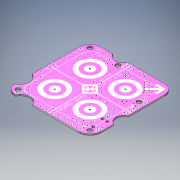
# Autodesk Inventor part: Eagle PCB rev 37
Saved by Autodesk Inventor 2016 (Build 200138000, 138)
## iProperties
Created: 2017-03-28
Part Number: Eagle PCB rev 37
Material: Generic
Document SubType Name: Modeling
Designer: Samuel Clay
Density: 1 g/cm^3
Appearance: Default
Author: Samuel Clay
Autodesk Inventor part; units mm, degrees
(part 1 of 2)
ref_plane "YZ Plane" through (0, 0, 0) normal (1, 0, 0) x (0, 1, 0)
ref_plane "XZ Plane" through (0, 0, 0) normal (0, 1, 0) x (-1, 0, 0)
ref_plane "XY Plane" through (0, 0, 0) normal (0, 0, 1) x (1, 0, 0)
sketch "PCB" plane through (0, 0, 0) normal (0, 0, 1) x (1, 0, 0)
  line L0 (-0.2705, -17.5177) -> (-0.2099, -17.5782)
  line L1 (0.0381, -17.435) -> (0.0159, -17.3523)
  line L2 (-0.2926, -17.435) -> (-0.2705, -17.5177)
  line L3 (-0.2099, -17.2918) -> (-0.2705, -17.3523)
  line L4 (-0.2705, -17.3523) -> (-0.2926, -17.435)
  line L5 (0.0159, -17.3523) -> (-0.0446, -17.2918)
  line L6 (-17.6003, -14.7625) -> (-17.5782, -14.8452)
  line L7 (-11.4091, 12.9967) -> (-11.4696, 12.9362)
  line L8 (-0.0446, -17.2918) -> (-0.1273, -17.2697)
  line L9 (-0.1273, -17.2697) -> (-0.2099, -17.2918)
  line L10 (-11.161, 12.8535) -> (-11.1832, 12.9362)
  line L11 (-0.2099, -17.5782) -> (-0.1273, -17.6003)
  line L12 (-11.2437, 12.9967) -> (-11.3264, 13.0189)
  line L13 (3.0162, 17.435) -> (3.0384, 17.3523)
  line L14 (-0.1273, -17.6003) -> (-0.0446, -17.5782)
  line L15 (-11.1832, 12.9362) -> (-11.2437, 12.9967)
  line L16 (-0.0446, -17.5782) -> (0.0159, -17.5177)
  line L17 (0.0159, -17.5177) -> (0.0381, -17.435)
  line L18 (-11.3264, 13.0189) -> (-11.4091, 12.9967)
  line L19 (-11.4696, 12.9362) -> (-11.4917, 12.8535)
  line L20 (-11.4917, 12.8535) -> (-11.4696, 12.7709)
  line L21 (-11.4696, 12.7709) -> (-11.4091, 12.7103)
  line L22 (-11.4091, 12.7103) -> (-11.3264, 12.6882)
  line L23 (-11.3264, 12.6882) -> (-11.2437, 12.7103)
  line L24 (-11.2437, 12.7103) -> (-11.1832, 12.7709)
  line L25 (-11.1832, 12.7709) -> (-11.161, 12.8535)
  line L26 (8.0176, -7.763) -> (7.9835, -7.6358)
  line L27 (7.9835, -7.6358) -> (7.8903, -7.5426)
  line L28 (7.8903, -7.5426) -> (7.763, -7.5085)
  line L29 (7.763, -7.5085) -> (7.6358, -7.5426)
  line L30 (7.6358, -7.5426) -> (7.5426, -7.6358)
  line L31 (7.5426, -7.6358) -> (7.5085, -7.763)
  line L32 (7.5085, -7.763) -> (7.5426, -7.8903)
  line L33 (7.5426, -7.8903) -> (7.6358, -7.9835)
  line L34 (7.6358, -7.9835) -> (7.763, -8.0176)
  line L35 (7.763, -8.0176) -> (7.8903, -7.9835)
  line L36 (7.8903, -7.9835) -> (7.9835, -7.8903)
  line L37 (7.9835, -7.8903) -> (8.0176, -7.763)
  line L38 (-18.2813, -15.6127) -> (-18.1967, -15.8611)
  line L39 (-13.3626, 15.4579) -> (-13.6171, 15.5261)
  line L40 (-6.9534, -18.4531) -> (13.3626, -18.4531)
  line L41 (-15.6051, -18.2836) -> (-15.3515, -18.3513)
  line L42 (14.9989, -18.1829) -> (15.3106, -18.0656)
  line L43 (-0.8082, 3.5474) -> (-0.7476, 3.6079)
  line L44 (-11.7528, 17.2918) -> (-11.6922, 17.3523)
  line L45 (-17.9797, -16.3387) -> (-17.8483, -16.5658)
  line L46 (16.719, -17.1898) -> (16.9621, -16.9621)
  line L47 (17.7711, -15.9078) -> (17.9281, -15.6141)
  line L48 (17.5782, -0.6809) -> (17.5177, -0.6204)
  line L49 (15.7965, -6.9168) -> (15.736, -6.8563)
  line L50 (17.5177, -0.6204) -> (17.435, -0.5982)
  line L51 (-14.2088, 17.2918) -> (-14.1262, 17.2697)
  line L52 (15.8187, -6.9995) -> (15.7965, -6.9168)
  line L53 (-13.983, 17.3523) -> (-13.9608, 17.435)
  line L54 (-14.2088, 17.5782) -> (-14.2694, 17.5177)
  line L55 (-14.2694, 17.5177) -> (-14.2915, 17.435)
  line L56 (-14.2915, 17.435) -> (-14.2694, 17.3523)
  line L57 (-14.2694, 17.3523) -> (-14.2088, 17.2918)
  line L58 (-0.7255, -15.3988) -> (-0.7476, -15.3161)
  line L59 (-13.983, 17.5177) -> (-14.0435, 17.5782)
  line L60 (-14.1262, 17.2697) -> (-14.0435, 17.2918)
  line L61 (-14.0435, 17.2918) -> (-13.983, 17.3523)
  line L62 (-14.1262, 17.6003) -> (-14.2088, 17.5782)
  line L63 (-13.9608, 17.435) -> (-13.983, 17.5177)
  line L64 (-14.0435, 17.5782) -> (-14.1262, 17.6003)
  line L65 (15.736, -6.8563) -> (15.6533, -6.8341)
  line L66 (-4.1997, -17.6003) -> (-4.117, -17.5782)
  line L67 (16.1624, -9.3283) -> (16.245, -9.3061)
  line L68 (17.435, -0.5982) -> (17.3523, -0.6204)
  line L69 (16.245, -9.3061) -> (16.3056, -9.2456)
  line L70 (-0.7476, -15.3161) -> (-0.8082, -15.2556)
  line L71 (-0.8082, -15.2556) -> (-0.8908, -15.2335)
  line L72 (-0.8908, -15.2335) -> (-0.9735, -15.2556)
  line L73 (-0.9735, -15.2556) -> (-1.034, -15.3161)
  line L74 (-1.034, -15.3161) -> (-1.0562, -15.3988)
  line L75 (-1.0562, -15.3988) -> (-1.034, -15.4815)
  line L76 (-1.034, -15.4815) -> (-0.9735, -15.542)
  line L77 (-0.9735, -15.542) -> (-0.8908, -15.5641)
  line L78 (-0.8908, -15.5641) -> (-0.8082, -15.542)
  line L79 (-0.8082, -15.542) -> (-0.7476, -15.4815)
  line L80 (-0.7476, -15.4815) -> (-0.7255, -15.3988)
  line L81 (8.1829, 15.1443) -> (8.1607, 15.2269)
  line L82 (-14.2375, 13.4453) -> (-14.298, 13.5058)
  line L83 (14.0435, -7.8744) -> (13.983, -7.9349)
  line L84 (13.983, -7.9349) -> (13.9608, -8.0176)
  line L85 (13.9608, -8.0176) -> (13.983, -8.1002)
  line L86 (13.983, -8.1002) -> (14.0435, -8.1607)
  line L87 (14.546, -10.8173) -> (14.5239, -10.7347)
  line L88 (14.5239, -10.7347) -> (14.4634, -10.6741)
  line L89 (14.2915, -8.0176) -> (14.2694, -7.9349)
  line L90 (14.4634, -10.6741) -> (14.3807, -10.652)
  line L91 (14.2694, -7.9349) -> (14.2088, -7.8744)
  line L92 (14.1262, -7.8522) -> (14.0435, -7.8744)
  line L93 (14.3807, -10.652) -> (14.298, -10.6741)
  line L94 (14.298, -10.6741) -> (14.2375, -10.7347)
  line L95 (14.2375, -10.7347) -> (14.2154, -10.8173)
  line L96 (14.2154, -10.8173) -> (14.2375, -10.9)
  line L97 (14.2375, -10.9) -> (14.298, -10.9605)
  line L98 (14.2088, -7.8744) -> (14.1262, -7.8522)
  line L99 (14.298, -10.9605) -> (14.3807, -10.9827)
  line L100 (14.0435, -8.1607) -> (14.1262, -8.1829)
  line L101 (14.3807, -10.9827) -> (14.4634, -10.9605)
  line L102 (14.4634, -10.9605) -> (14.5239, -10.9)
  line L103 (14.5239, -10.9) -> (14.546, -10.8173)
  line L104 (14.1262, -8.1829) -> (14.2088, -8.1607)
  line L105 (14.2088, -8.1607) -> (14.2694, -8.1002)
  line L106 (14.2694, -8.1002) -> (14.2915, -8.0176)
  line L107 (-14.298, 13.5058) -> (-14.3807, 13.5279)
  line L108 (-14.3807, 13.5279) -> (-14.4634, 13.5058)
  line L109 (13.5058, -15.0616) -> (13.4453, -15.0011)
  line L110 (16.3056, -0.5536) -> (16.245, -0.4931)
  line L111 (-18.4531, 13.3626) -> (-18.4531, -6.6988)
  line L112 (-17.7589, -7.0832) -> (-18.0967, -6.8742)
  line L113 (-16.8879, -7.8911) -> (-17.1517, -7.5941)
  line L114 (16.0192, -0.5536) -> (15.997, -0.6363)
  line L115 (-16.6541, -8.2122) -> (-16.8879, -7.8911)
  line L116 (-16.2848, -8.9145) -> (-16.4524, -8.5544)
  line L117 (-16.1527, -9.2892) -> (-16.2848, -8.9145)
  line L118 (16.245, -0.4931) -> (16.1624, -0.471)
  line L119 (-16.4524, -8.5544) -> (-16.6541, -8.2122)
  line L120 (2.5612, 11.9181) -> (2.5007, 11.9786)
  line L121 (-17.4429, -7.3239) -> (-17.7589, -7.0832)
  line L122 (-8.2721, 15.5943) -> (-8.0858, 15.7806)
  line L123 (-17.1517, -7.5941) -> (-17.4429, -7.3239)
  line L124 (-16.6541, -12.717) -> (-16.4524, -12.3748)
  line L125 (-8.0858, 15.7806) -> (-8.0176, 16.0351)
  line L126 (-18.0967, -6.8742) -> (-18.4531, -6.6988)
  line L127 (-16.0575, -9.6748) -> (-16.1527, -9.2892)
  line L128 (16.1624, -0.471) -> (16.0797, -0.4931)
  line L129 (-16, -10.0678) -> (-16.0575, -9.6748)
  line L130 (16.0797, -0.4931) -> (16.0192, -0.5536)
  line L131 (-15.9808, -10.4646) -> (-16, -10.0678)
  line L132 (-16, -10.8614) -> (-15.9808, -10.4646)
  line L133 (-8.0176, 13.9989) -> (-8.0858, 14.2534)
  line L134 (-16.0575, -11.2544) -> (-16, -10.8614)
  line L135 (-16.1527, -11.6401) -> (-16.0575, -11.2544)
  line L136 (15.997, -0.6363) -> (16.0192, -0.719)
  line L137 (-16.2848, -12.0147) -> (-16.1527, -11.6401)
  line L138 (-16.4524, -12.3748) -> (-16.2848, -12.0147)
  line L139 (16.0192, -0.719) -> (16.0797, -0.7795)
  line L140 (-8.9675, 14.2534) -> (-9.0357, 13.9989)
  line L141 (-16.8879, -13.0381) -> (-16.6541, -12.717)
  line L142 (16.0797, -0.7795) -> (16.1624, -0.8017)
  line L143 (-17.1517, -13.3351) -> (-16.8879, -13.0381)
  line L144 (-8.0858, 14.2534) -> (-8.2721, 14.4398)
  line L145 (-17.4429, -13.6053) -> (-17.1517, -13.3351)
  line L146 (16.3277, -0.6363) -> (16.3056, -0.5536)
  line L147 (16.1624, -0.8017) -> (16.245, -0.7795)
  line L148 (-17.7589, -13.846) -> (-17.4429, -13.6053)
  line L149 (-8.2721, 14.4398) -> (-8.5266, 14.508)
  line L150 (-18.0967, -14.055) -> (-17.7589, -13.846)
  line L151 (16.245, -0.7795) -> (16.3056, -0.719)
  line L152 (-18.4531, -14.2304) -> (-18.0967, -14.055)
  line L153 (15.6533, -6.8341) -> (15.5706, -6.8563)
  line L154 (16.3056, -0.719) -> (16.3277, -0.6363)
  line L155 (-18.4528, -14.5799) -> (-18.4354, -14.8417)
  line L156 (-8.5266, 14.508) -> (-8.7811, 14.4398)
  line L157 (-18.4354, -14.8417) -> (-18.4009, -15.1019)
  line L158 (-18.4009, -15.1019) -> (-18.3495, -15.3592)
  line L159 (-8.7811, 14.4398) -> (-8.9675, 14.2534)
  line L160 (-18.3495, -15.3592) -> (-18.2813, -15.6127)
  line L161 (-18.1967, -15.8611) -> (-18.096, -16.1034)
  line L162 (-18.096, -16.1034) -> (-17.9797, -16.3387)
  line L163 (-7.5426, 7.6358) -> (-7.5085, 7.763)
  line L164 (-9.1788, -14.8071) -> (-9.201, -14.8897)
  line L165 (-17.8483, -16.5658) -> (-17.7023, -16.7839)
  line L166 (-17.7023, -16.7839) -> (-17.5423, -16.9919)
  line L167 (-17.5423, -16.9919) -> (-17.3691, -17.1891)
  line L168 (-17.3691, -17.1891) -> (-17.1833, -17.3745)
  line L169 (-17.1833, -17.3745) -> (-16.9858, -17.5473)
  line L170 (-16.9858, -17.5473) -> (-16.7775, -17.7069)
  line L171 (-16.7775, -17.7069) -> (-16.5591, -17.8524)
  line L172 (-16.5591, -17.8524) -> (-16.3317, -17.9834)
  line L173 (-16.3317, -17.9834) -> (-16.0962, -18.0993)
  line L174 (-16.0962, -18.0993) -> (-15.8537, -18.1995)
  line L175 (-15.8537, -18.1995) -> (-15.6051, -18.2836)
  line L176 (-15.3515, -18.3513) -> (-15.0941, -18.4022)
  line L177 (-15.0941, -18.4022) -> (-14.8339, -18.4362)
  line L178 (-14.8339, -18.4362) -> (-14.572, -18.4531)
  line L179 (-14.572, -18.4531) -> (-14.4849, -18.4531)
  line L180 (-14.3095, -18.0967) -> (-14.4849, -18.4531)
  line L181 (-14.1005, -17.7589) -> (-14.3095, -18.0967)
  line L182 (-13.8598, -17.4429) -> (-14.1005, -17.7589)
  line L183 (-13.5897, -17.1517) -> (-13.8598, -17.4429)
  line L184 (-13.2927, -16.8879) -> (-13.5897, -17.1517)
  line L185 (-2.5898, 3.5474) -> (-2.5293, 3.6079)
  line L186 (-12.9715, -16.6541) -> (-13.2927, -16.8879)
  line L187 (-2.6725, 3.5253) -> (-2.5898, 3.5474)
  line L188 (-12.6293, -16.4524) -> (-12.9715, -16.6541)
  line L189 (-12.2692, -16.2848) -> (-12.6293, -16.4524)
  line L190 (-11.8946, -16.1527) -> (-12.2692, -16.2848)
  line L191 (-11.5089, -16.0575) -> (-11.8946, -16.1527)
  line L192 (-11.1159, -16) -> (-11.5089, -16.0575)
  line L193 (-10.7191, -15.9808) -> (-11.1159, -16)
  line L194 (-10.3224, -16) -> (-10.7191, -15.9808)
  line L195 (-9.9293, -16.0575) -> (-10.3224, -16)
  line L196 (-9.5437, -16.1527) -> (-9.9293, -16.0575)
  line L197 (-9.1691, -16.2848) -> (-9.5437, -16.1527)
  line L198 (-8.8089, -16.4524) -> (-9.1691, -16.2848)
  line L199 (-8.4667, -16.6541) -> (-8.8089, -16.4524)
  line L200 (-8.1456, -16.8879) -> (-8.4667, -16.6541)
  line L201 (-7.8486, -17.1517) -> (-8.1456, -16.8879)
  line L202 (-7.5785, -17.4429) -> (-7.8486, -17.1517)
  line L203 (-7.3378, -17.7589) -> (-7.5785, -17.4429)
  line L204 (-7.1287, -18.0967) -> (-7.3378, -17.7589)
  line L205 (-6.9534, -18.4531) -> (-7.1287, -18.0967)
  line L206 (13.3626, -18.4531) -> (13.6955, -18.4422)
  line L207 (13.6955, -18.4422) -> (14.027, -18.4095)
  line L208 (14.027, -18.4095) -> (14.3557, -18.3553)
  line L209 (14.3557, -18.3553) -> (14.6801, -18.2796)
  line L210 (14.6801, -18.2796) -> (14.9989, -18.1829)
  line L211 (15.3106, -18.0656) -> (15.6141, -17.9281)
  line L212 (15.6141, -17.9281) -> (15.9078, -17.7711)
  line L213 (15.9078, -17.7711) -> (16.1907, -17.5952)
  line L214 (16.1907, -17.5952) -> (16.4615, -17.4012)
  line L215 (16.4615, -17.4012) -> (16.719, -17.1898)
  line L216 (16.9621, -16.9621) -> (17.1898, -16.719)
  line L217 (17.1898, -16.719) -> (17.4012, -16.4615)
  line L218 (17.4012, -16.4615) -> (17.5952, -16.1907)
  line L219 (17.5952, -16.1907) -> (17.7711, -15.9078)
  line L220 (17.9281, -15.6141) -> (18.0656, -15.3106)
  line L221 (-2.5293, 3.6079) -> (-2.5072, 3.6906)
  line L222 (18.0656, -15.3106) -> (18.1829, -14.9989)
  line L223 (18.1829, -14.9989) -> (18.2796, -14.6801)
  line L224 (18.2796, -14.6801) -> (18.3553, -14.3557)
  line L225 (18.3553, -14.3557) -> (18.4095, -14.027)
  line L226 (18.4095, -14.027) -> (18.4422, -13.6955)
  line L227 (18.4422, -13.6955) -> (18.4531, -13.3626)
  line L228 (18.4531, -13.3626) -> (18.4531, -8.3763)
  line L229 (18.1449, -8.2246) -> (18.4531, -8.3763)
  line L230 (17.8528, -8.0438) -> (18.1449, -8.2246)
  line L231 (17.5795, -7.8357) -> (17.8528, -8.0438)
  line L232 (17.3276, -7.6021) -> (17.5795, -7.8357)
  line L233 (17.0995, -7.3452) -> (17.3276, -7.6021)
  line L234 (16.8973, -7.0675) -> (17.0995, -7.3452)
  line L235 (16.7229, -6.7715) -> (16.8973, -7.0675)
  line L236 (16.5779, -6.4601) -> (16.7229, -6.7715)
  line L237 (16.4637, -6.1361) -> (16.5779, -6.4601)
  line L238 (16.3813, -5.8026) -> (16.4637, -6.1361)
  line L239 (16.3316, -5.4627) -> (16.3813, -5.8026)
  line L240 (16.315, -5.1196) -> (16.3316, -5.4627)
  line L241 (16.3316, -4.7764) -> (16.315, -5.1196)
  line L242 (16.3813, -4.4365) -> (16.3316, -4.7764)
  line L243 (16.4637, -4.103) -> (16.3813, -4.4365)
  line L244 (16.5779, -3.779) -> (16.4637, -4.103)
  line L245 (16.7229, -3.4676) -> (16.5779, -3.779)
  line L246 (16.8973, -3.1716) -> (16.7229, -3.4676)
  line L247 (17.0995, -2.8939) -> (16.8973, -3.1716)
  line L248 (17.3276, -2.6371) -> (17.0995, -2.8939)
  line L249 (17.5795, -2.4035) -> (17.3276, -2.6371)
  line L250 (17.8528, -2.1953) -> (17.5795, -2.4035)
  line L251 (18.1449, -2.0145) -> (17.8528, -2.1953)
  line L252 (18.4531, -1.8628) -> (18.1449, -2.0145)
  line L253 (18.4531, -1.8628) -> (18.4531, 14.3807)
  line L254 (18.4531, 14.3807) -> (18.4444, 14.647)
  line L255 (18.4444, 14.647) -> (18.4183, 14.9122)
  line L256 (18.4183, 14.9122) -> (18.3748, 15.1752)
  line L257 (18.3748, 15.1752) -> (18.3143, 15.4347)
  line L258 (18.3143, 15.4347) -> (18.237, 15.6897)
  line L259 (18.237, 15.6897) -> (18.1431, 15.9391)
  line L260 (18.1431, 15.9391) -> (18.0331, 16.1819)
  line L261 (18.0331, 16.1819) -> (17.9075, 16.4169)
  line L262 (17.9075, 16.4169) -> (17.7668, 16.6432)
  line L263 (17.7668, 16.6432) -> (17.6116, 16.8598)
  line L264 (17.6116, 16.8598) -> (17.4425, 17.0658)
  line L265 (17.4425, 17.0658) -> (17.2603, 17.2603)
  line L266 (17.2603, 17.2603) -> (17.0658, 17.4425)
  line L267 (17.0658, 17.4425) -> (16.8598, 17.6116)
  line L268 (16.8598, 17.6116) -> (16.6432, 17.7668)
  line L269 (16.6432, 17.7668) -> (16.4169, 17.9075)
  line L270 (16.4169, 17.9075) -> (16.1819, 18.0331)
  line L271 (16.1819, 18.0331) -> (15.9391, 18.1431)
  line L272 (15.9391, 18.1431) -> (15.6897, 18.237)
  line L273 (15.6897, 18.237) -> (15.4347, 18.3143)
  line L274 (15.4347, 18.3143) -> (15.1752, 18.3749)
  line L275 (15.1752, 18.3749) -> (14.9122, 18.4183)
  line L276 (14.9122, 18.4183) -> (14.647, 18.4444)
  line L277 (14.647, 18.4444) -> (14.3807, 18.4531)
  line L278 (14.3807, 18.4531) -> (-1.6083, 18.4531)
  line L279 (-1.76, 18.1449) -> (-1.6083, 18.4531)
  line L280 (-1.9408, 17.8528) -> (-1.76, 18.1449)
  line L281 (-2.1489, 17.5795) -> (-1.9408, 17.8528)
  line L282 (-18.0656, 15.3106) -> (-18.1829, 14.9989)
  line L283 (-12.7103, 17.5177) -> (-12.7709, 17.5782)
  line L284 (-15.3988, -16.535) -> (-15.0261, -16.1624)
  line L285 (14.492, 2.3353) -> (14.5525, 2.2748)
  line L286 (16.026, -3.4361) -> (16.1624, -2.927)
  line L287 (-9.0357, 17.6003) -> (-9.1183, 17.5782)
  line L288 (1.8198, -17.435) -> (1.7976, -17.3523)
  line L289 (-17.5952, 16.1907) -> (-17.7711, 15.9078)
  line L290 (-14.6801, 18.2796) -> (-14.9989, 18.1829)
  line L291 (15.1443, -16.535) -> (15.6533, -16.6714)
  line L292 (-5.3291, 14.0816) -> (-5.3896, 14.1421)
  line L293 (15.6533, -16.6714) -> (16.1624, -16.535)
  line L294 (11.4696, 12.5163) -> (11.4917, 12.599)
  line L295 (16.1624, -16.535) -> (16.535, -16.1624)
  line L296 (-6.5731, 14.1102) -> (-6.4904, 14.0881)
  line L297 (16.535, -16.1624) -> (16.6714, -15.6533)
  line L298 (10.4196, 15.4815) -> (10.3975, 15.3988)
  line L299 (16.7828, 7.044) -> (16.8433, 6.9835)
  line L300 (-6.4904, 14.0881) -> (-6.4077, 14.1102)
  line L301 (10.7282, 15.3988) -> (10.706, 15.4815)
  line L302 (10.6455, 13.2513) -> (10.5628, 13.2734)
  line L303 (13.2194, 2.0808) -> (13.2799, 2.0203)
  line L304 (5.0996, 15.1443) -> (5.4723, 14.7716)
  line L305 (5.9813, 16.6714) -> (5.4723, 16.535)
  line L306 (5.4723, 16.535) -> (5.0996, 16.1624)
  line L307 (17.0691, 7.2094) -> (17.0086, 7.2699)
  line L308 (5.0996, 16.1624) -> (4.9632, 15.6533)
  line L309 (4.9632, 15.6533) -> (5.0996, 15.1443)
  line L310 (-6.6557, 14.2534) -> (-6.6336, 14.1708)
  line L311 (11.161, 12.599) -> (11.1832, 12.5163)
  line L312 (5.4723, 14.7716) -> (5.9813, 14.6352)
  line L313 (6.4904, 16.535) -> (5.9813, 16.6714)
  line L314 (5.9813, 14.6352) -> (6.4904, 14.7716)
  line L315 (-6.4904, 14.4188) -> (-6.5731, 14.3966)
  line L316 (6.4904, 14.7716) -> (6.8631, 15.1443)
  line L317 (10.4196, 13.0254) -> (10.4801, 12.9649)
  line L318 (6.9995, 15.6533) -> (6.8631, 16.1624)
  line L319 (6.8631, 15.1443) -> (6.9995, 15.6533)
  line L320 (10.706, 13.1907) -> (10.6455, 13.2513)
  line L321 (12.3286, 11.371) -> (12.3891, 11.3105)
  line L322 (12.4718, 11.619) -> (12.3891, 11.5968)
  line L323 (10.6455, 15.542) -> (10.5628, 15.5641)
  line L324 (10.4801, 12.9649) -> (10.5628, 12.9427)
  line L325 (11.2437, 12.7422) -> (11.1832, 12.6817)
  line L326 (11.4696, 12.6817) -> (11.4091, 12.7422)
  line L327 (13.2194, -17.3523) -> (13.1972, -17.435)
  line L328 (13.2799, -17.2918) -> (13.2194, -17.3523)
  line L329 (6.8631, 16.1624) -> (6.4904, 16.535)
  line L330 (11.4091, 12.4558) -> (11.4696, 12.5163)
  line L331 (4.117, 15.0011) -> (4.1997, 14.9789)
  line L332 (11.4917, 12.599) -> (11.4696, 12.6817)
  line L333 (11.3264, 12.4337) -> (11.4091, 12.4558)
  line L334 (-5.3896, 13.8557) -> (-5.3291, 13.9162)
  line L335 (11.2437, 12.4558) -> (11.3264, 12.4337)
  line L336 (-6.5731, 14.3966) -> (-6.6336, 14.3361)
  line L337 (4.3429, 15.2269) -> (4.2823, 15.2875)
  line L338 (13.3626, -17.2697) -> (13.2799, -17.2918)
  line L339 (-11.8354, 17.2697) -> (-11.7528, 17.2918)
  line L340 (-6.6336, 14.3361) -> (-6.6557, 14.2534)
  line L341 (4.3429, 15.0616) -> (4.365, 15.1443)
  line L342 (-5.3291, 13.9162) -> (-5.307, 13.9989)
  line L343 (-12.9362, 17.2918) -> (-12.8535, 17.2697)
  line L344 (-17.2697, -4.1997) -> (-17.2918, -4.117)
  line L345 (13.5279, -17.435) -> (13.5058, -17.3523)
  line L346 (13.5058, -17.3523) -> (13.4453, -17.2918)
  line L347 (-6.3472, 14.1708) -> (-6.3251, 14.2534)
  line L348 (17.0913, 7.1267) -> (17.0691, 7.2094)
  line L349 (-11.8354, 17.6003) -> (-11.9181, 17.5782)
  line L350 (-6.3472, 14.3361) -> (-6.4077, 14.3966)
  line L351 (10.7282, 13.1081) -> (10.706, 13.1907)
  line L352 (-5.555, 14.1421) -> (-5.6155, 14.0816)
  line L353 (16.8433, 7.2699) -> (16.7828, 7.2094)
  line L354 (17.0086, 7.2699) -> (16.9259, 7.2921)
  line L355 (-5.6155, 14.0816) -> (-5.6376, 13.9989)
  line L356 (11.4091, 12.7422) -> (11.3264, 12.7644)
  line L357 (-5.6155, 13.9162) -> (-5.555, 13.8557)
  line L358 (-6.4077, 14.3966) -> (-6.4904, 14.4188)
  line L359 (-5.3896, 14.1421) -> (-5.4723, 14.1642)
  line L360 (10.4196, 15.3161) -> (10.4801, 15.2556)
  line L361 (10.4801, 15.2556) -> (10.5628, 15.2335)
  line L362 (11.1832, 12.6817) -> (11.161, 12.599)
  line L363 (11.3264, 12.7644) -> (11.2437, 12.7422)
  line L364 (16.9259, 6.9614) -> (17.0086, 6.9835)
  line L365 (17.0691, 7.044) -> (17.0913, 7.1267)
  line L366 (10.4196, 13.1907) -> (10.3975, 13.1081)
  line L367 (12.6371, 11.4536) -> (12.6149, 11.5363)
  line L368 (10.3975, 13.1081) -> (10.4196, 13.0254)
  line L369 (13.2799, 2.0203) -> (13.3626, 1.9981)
  line L370 (16.8433, 6.9835) -> (16.9259, 6.9614)
  line L371 (17.0086, 6.9835) -> (17.0691, 7.044)
  line L372 (10.5628, 12.9427) -> (10.6455, 12.9649)
  line L373 (10.6455, 12.9649) -> (10.706, 13.0254)
  line L374 (10.706, 13.0254) -> (10.7282, 13.1081)
  line L375 (12.4718, 11.2883) -> (12.5544, 11.3105)
  line L376 (12.5544, 11.3105) -> (12.6149, 11.371)
  line L377 (12.6149, 11.371) -> (12.6371, 11.4536)
  line L378 (16.9259, 7.2921) -> (16.8433, 7.2699)
  line L379 (10.3975, 15.3988) -> (10.4196, 15.3161)
  line L380 (16.7606, 7.1267) -> (16.7828, 7.044)
  line L381 (10.5628, 15.2335) -> (10.6455, 15.2556)
  line L382 (10.6455, 15.2556) -> (10.706, 15.3161)
  line L383 (10.706, 15.3161) -> (10.7282, 15.3988)
  line L384 (10.706, 15.4815) -> (10.6455, 15.542)
  line L385 (4.0565, 15.2269) -> (4.0343, 15.1443)
  line L386 (10.5628, 15.5641) -> (10.4801, 15.542)
  line L387 (10.4801, 15.542) -> (10.4196, 15.4815)
  line L388 (4.0343, 15.1443) -> (4.0565, 15.0616)
  line L389 (4.0565, 15.0616) -> (4.117, 15.0011)
  line L390 (12.3286, 11.5363) -> (12.3064, 11.4536)
  line L391 (12.3064, 11.4536) -> (12.3286, 11.371)
  line L392 (12.3891, 11.3105) -> (12.4718, 11.2883)
  line L393 (11.7241, 14.4634) -> (11.6636, 14.5239)
  line L394 (11.6636, 14.5239) -> (11.5809, 14.546)
  line L395 (11.4377, 14.298) -> (11.4982, 14.2375)
  line L396 (11.5809, 14.546) -> (11.4982, 14.5239)
  line L397 (11.4982, 14.5239) -> (11.4377, 14.4634)
  line L398 (3.0384, 1.699) -> (3.0989, 1.6385)
  line L399 (-6.3251, 14.2534) -> (-6.3472, 14.3361)
  line L400 (11.4377, 14.4634) -> (11.4156, 14.3807)
  line L401 (11.4156, 14.3807) -> (11.4377, 14.298)
  line L402 (11.7463, 14.3807) -> (11.7241, 14.4634)
  line L403 (11.4982, 14.2375) -> (11.5809, 14.2154)
  line L404 (11.5809, 14.2154) -> (11.6636, 14.2375)
  line L405 (11.6636, 14.2375) -> (11.7241, 14.298)
  line L406 (11.7241, 14.298) -> (11.7463, 14.3807)
  line L407 (12.6371, 13.4899) -> (12.6149, 13.5725)
  line L408 (16.7828, 7.2094) -> (16.7606, 7.1267)
  line L409 (-2.5007, 14.9057) -> (-2.5612, 14.8452)
  line L410 (4.1997, 14.9789) -> (4.2823, 15.0011)
  line L411 (12.6149, 13.5725) -> (12.5544, 13.633)
  line L412 (12.5544, 13.633) -> (12.4718, 13.6552)
  line L413 (4.117, 15.2875) -> (4.0565, 15.2269)
  line L414 (12.4718, 13.6552) -> (12.3891, 13.633)
  line L415 (12.3891, 13.633) -> (12.3286, 13.5725)
  line L416 (12.3286, 13.5725) -> (12.3064, 13.4899)
  line L417 (4.1997, 15.3096) -> (4.117, 15.2875)
  line L418 (3.1816, 1.947) -> (3.0989, 1.9249)
  line L419 (12.3064, 13.4899) -> (12.3286, 13.4072)
  line L420 (4.2823, 15.2875) -> (4.1997, 15.3096)
  line L421 (12.3286, 13.4072) -> (12.3891, 13.3467)
  line L422 (12.3891, 13.3467) -> (12.4718, 13.3245)
  line L423 (12.4718, 13.3245) -> (12.5544, 13.3467)
  line L424 (12.5544, 13.3467) -> (12.6149, 13.4072)
  line L425 (12.6149, 13.4072) -> (12.6371, 13.4899)
  line L426 (12.3891, 11.5968) -> (12.3286, 11.5363)
  line L427 (13.1972, -17.435) -> (13.2194, -17.5177)
  line L428 (4.365, 15.1443) -> (4.3429, 15.2269)
  line L429 (3.0989, 1.6385) -> (3.1816, 1.6163)
  line L430 (3.1816, 1.6163) -> (3.2642, 1.6385)
  line L431 (13.2194, -17.5177) -> (13.2799, -17.5782)
  line L432 (8.5712, -14.0148) -> (8.6539, -14.037)
  line L433 (13.2799, -17.5782) -> (13.3626, -17.6003)
  line L434 (13.3626, -17.6003) -> (13.4453, -17.5782)
  line L435 (13.4453, -17.5782) -> (13.5058, -17.5177)
  line L436 (13.5058, -17.5177) -> (13.5279, -17.435)
  line L437 (8.5107, -13.9543) -> (8.5712, -14.0148)
  line L438 (-2.3353, 14.9057) -> (-2.418, 14.9278)
  line L439 (13.4453, -17.2918) -> (13.3626, -17.2697)
  line L440 (-2.3353, 14.6193) -> (-2.2748, 14.6798)
  line L441 (-2.418, 14.9278) -> (-2.5007, 14.9057)
  line L442 (-2.2527, 14.7625) -> (-2.2748, 14.8452)
  line L443 (8.7971, -13.9543) -> (8.8192, -13.8716)
  line L444 (8.7365, -14.0148) -> (8.7971, -13.9543)
  line L445 (11.2372, -17.435) -> (11.215, -17.3523)
  line L446 (11.215, -17.3523) -> (11.1545, -17.2918)
  line L447 (11.1545, -17.2918) -> (11.0719, -17.2697)
  line L448 (8.5107, -13.789) -> (8.4885, -13.8716)
  line L449 (10.9287, -17.5177) -> (10.9892, -17.5782)
  line L450 (11.0719, -17.2697) -> (10.9892, -17.2918)
  line L451 (8.8192, -13.8716) -> (8.7971, -13.789)
  line L452 (10.9892, -17.2918) -> (10.9287, -17.3523)
  line L453 (10.9287, -17.3523) -> (10.9065, -17.435)
  line L454 (10.9065, -17.435) -> (10.9287, -17.5177)
  line L455 (10.9892, -17.5782) -> (11.0719, -17.6003)
  line L456 (-2.2748, 14.8452) -> (-2.3353, 14.9057)
  line L457 (11.0719, -17.6003) -> (11.1545, -17.5782)
  line L458 (8.4885, -13.8716) -> (8.5107, -13.9543)
  line L459 (11.1545, -17.5782) -> (11.215, -17.5177)
  line L460 (8.7365, -13.7285) -> (8.6539, -13.7063)
  line L461 (11.215, -17.5177) -> (11.2372, -17.435)
  line L462 (8.9243, -17.5177) -> (8.9465, -17.435)
  line L463 (-2.418, 14.5971) -> (-2.3353, 14.6193)
  line L464 (-2.2748, 14.6798) -> (-2.2527, 14.7625)
  line L465 (8.5712, -13.7285) -> (8.5107, -13.789)
  line L466 (-2.5612, 14.6798) -> (-2.5007, 14.6193)
  line L467 (-2.5007, 14.6193) -> (-2.418, 14.5971)
  line L468 (8.9465, -17.435) -> (8.9243, -17.3523)
  line L469 (8.9243, -17.3523) -> (8.8638, -17.2918)
  line L470 (8.6539, -14.037) -> (8.7365, -14.0148)
  line L471 (8.8638, -17.2918) -> (8.7811, -17.2697)
  line L472 (8.7811, -17.2697) -> (8.6985, -17.2918)
  line L473 (8.6985, -17.2918) -> (8.6379, -17.3523)
  line L474 (-7.6358, 7.5426) -> (-7.5426, 7.6358)
  line L475 (8.6379, -17.3523) -> (8.6158, -17.435)
  line L476 (8.6539, -13.7063) -> (8.5712, -13.7285)
  line L477 (8.6158, -17.435) -> (8.6379, -17.5177)
  line L478 (8.6379, -17.5177) -> (8.6985, -17.5782)
  line L479 (8.6985, -17.5782) -> (8.7811, -17.6003)
  line L480 (8.7811, -17.6003) -> (8.8638, -17.5782)
  line L481 (8.8638, -17.5782) -> (8.9243, -17.5177)
  line L482 (8.7971, -13.789) -> (8.7365, -13.7285)
  line L483 (-2.5833, 14.7625) -> (-2.5612, 14.6798)
  line L484 (-2.5612, 14.8452) -> (-2.5833, 14.7625)
  line L485 (-4.0343, -17.435) -> (-4.0565, -17.3523)
  line L486 (-4.0565, -17.3523) -> (-4.117, -17.2918)
  line L487 (-4.117, -17.2918) -> (-4.1997, -17.2697)
  line L488 (-4.1997, -17.2697) -> (-4.2823, -17.2918)
  line L489 (-4.3429, -17.5177) -> (-4.2823, -17.5782)
  line L490 (-4.2823, -17.2918) -> (-4.3429, -17.3523)
  line L491 (-4.3429, -17.3523) -> (-4.365, -17.435)
  line L492 (-4.365, -17.435) -> (-4.3429, -17.5177)
  line L493 (-4.2823, -17.5782) -> (-4.1997, -17.6003)
  line L494 (-17.2697, -14.7625) -> (-17.2918, -14.6798)
  line L495 (17.3523, 1.384) -> (17.435, 1.3618)
  line L496 (17.5177, 1.384) -> (17.5782, 1.4445)
  line L497 (-17.2918, -14.6798) -> (-17.3523, -14.6193)
  line L498 (-17.3523, -14.6193) -> (-17.435, -14.5971)
  line L499 (17.435, 1.3618) -> (17.5177, 1.384)
  line L500 (-17.435, -4.0343) -> (-17.5177, -4.0565)
  line L501 (-17.2918, -4.117) -> (-17.3523, -4.0565)
  line L502 (-17.5177, -4.0565) -> (-17.5782, -4.117)
  line L503 (-17.5782, -4.117) -> (-17.6003, -4.1997)
  line L504 (-17.6003, -4.1997) -> (-17.5782, -4.2823)
  line L505 (-17.5782, -4.2823) -> (-17.5177, -4.3429)
  line L506 (-17.5177, -4.3429) -> (-17.435, -4.365)
  line L507 (-17.435, -4.365) -> (-17.3523, -4.3429)
  line L508 (-17.3523, -4.3429) -> (-17.2918, -4.2823)
  line L509 (-17.2918, -4.2823) -> (-17.2697, -4.1997)
  line L510 (3.3248, 17.5177) -> (3.2642, 17.5782)
  line L511 (-17.3523, -4.0565) -> (-17.435, -4.0343)
  line L512 (3.1816, 17.2697) -> (3.2642, 17.2918)
  line L513 (3.2642, 17.2918) -> (3.3248, 17.3523)
  line L514 (3.2642, 17.5782) -> (3.1816, 17.6003)
  line L515 (3.3248, 17.3523) -> (3.3469, 17.435)
  line L516 (3.0384, 17.3523) -> (3.0989, 17.2918)
  line L517 (3.1816, 17.6003) -> (3.0989, 17.5782)
  line L518 (3.0989, 17.2918) -> (3.1816, 17.2697)
  line L519 (3.3469, 17.435) -> (3.3248, 17.5177)
  line L520 (3.0384, 17.5177) -> (3.0162, 17.435)
  line L521 (3.0989, 17.5782) -> (3.0384, 17.5177)
  line L522 (12.5544, 11.5968) -> (12.4718, 11.619)
  line L523 (17.435, -0.9289) -> (17.5177, -0.9068)
  line L524 (12.6149, 11.5363) -> (12.5544, 11.5968)
  line L525 (17.2918, -0.8462) -> (17.3523, -0.9068)
  line L526 (17.3523, -0.9068) -> (17.435, -0.9289)
  line L527 (17.2697, -0.7636) -> (17.2918, -0.8462)
  line L528 (17.5177, -0.9068) -> (17.5782, -0.8462)
  line L529 (17.3523, -0.6204) -> (17.2918, -0.6809)
  line L530 (17.2918, -0.6809) -> (17.2697, -0.7636)
  line L531 (17.5782, -0.8462) -> (17.6003, -0.7636)
  line L532 (17.6003, -0.7636) -> (17.5782, -0.6809)
  line L533 (-1.8709, 12.8535) -> (-1.893, 12.9362)
  line L534 (-1.893, 12.9362) -> (-1.9535, 12.9967)
  line L535 (-1.9535, 12.9967) -> (-2.0362, 13.0189)
  line L536 (-2.0362, 13.0189) -> (-2.1189, 12.9967)
  line L537 (-2.1189, 12.9967) -> (-2.1794, 12.9362)
  line L538 (13.7825, -5.9813) -> (13.7603, -5.8987)
  line L539 (13.7603, -5.8987) -> (13.6998, -5.8382)
  line L540 (13.6998, -5.8382) -> (13.6171, -5.816)
  line L541 (13.6171, -5.816) -> (13.5344, -5.8382)
  line L542 (13.4739, -6.064) -> (13.5344, -6.1245)
  line L543 (13.5344, -5.8382) -> (13.4739, -5.8987)
  line L544 (13.4739, -5.8987) -> (13.4518, -5.9813)
  line L545 (13.4518, -5.9813) -> (13.4739, -6.064)
  line L546 (13.5344, -6.1245) -> (13.6171, -6.1467)
  line L547 (13.6171, -6.1467) -> (13.6998, -6.1245)
  line L548 (13.6998, -6.1245) -> (13.7603, -6.064)
  line L549 (13.7603, -6.064) -> (13.7825, -5.9813)
  line L550 (-14.9343, 9.147) -> (-14.8738, 9.2075)
  line L551 (-13.3245, 16.6714) -> (-13.3467, 16.7541)
  line L552 (-13.3467, 16.7541) -> (-13.4072, 16.8146)
  line L553 (-13.4072, 16.8146) -> (-13.4899, 16.8368)
  line L554 (-13.4899, 16.8368) -> (-13.5725, 16.8146)
  line L555 (-13.633, 16.5888) -> (-13.5725, 16.5282)
  line L556 (-13.5725, 16.8146) -> (-13.633, 16.7541)
  line L557 (-13.633, 16.7541) -> (-13.6552, 16.6714)
  line L558 (-13.6552, 16.6714) -> (-13.633, 16.5888)
  line L559 (-13.5725, 16.5282) -> (-13.4899, 16.5061)
  line L560 (-13.4899, 16.5061) -> (-13.4072, 16.5282)
  line L561 (-13.4072, 16.5282) -> (-13.3467, 16.5888)
  line L562 (-13.3467, 16.5888) -> (-13.3245, 16.6714)
  line L563 (5.0013, -14.3807) -> (4.9792, -14.298)
  line L564 (4.9792, -14.298) -> (4.9187, -14.2375)
  line L565 (4.9187, -14.2375) -> (4.836, -14.2154)
  line L566 (4.836, -14.2154) -> (4.7533, -14.2375)
  line L567 (4.7533, -14.2375) -> (4.6928, -14.298)
  line L568 (4.6928, -14.298) -> (4.6706, -14.3807)
  line L569 (-13.07, 10.5628) -> (-13.0921, 10.6455)
  line L570 (-13.0921, 10.6455) -> (-13.1527, 10.706)
  line L571 (-13.1527, 10.706) -> (-13.2353, 10.7282)
  line L572 (-13.2353, 10.7282) -> (-13.318, 10.706)
  line L573 (-13.318, 10.706) -> (-13.3785, 10.6455)
  line L574 (-13.3785, 10.6455) -> (-13.4007, 10.5628)
  line L575 (-13.4007, 10.5628) -> (-13.3785, 10.4801)
  line L576 (-13.3785, 10.4801) -> (-13.318, 10.4196)
  line L577 (-13.318, 10.4196) -> (-13.2353, 10.3975)
  line L578 (-13.2353, 10.3975) -> (-13.1527, 10.4196)
  line L579 (-13.1527, 10.4196) -> (-13.0921, 10.4801)
  line L580 (-13.0921, 10.4801) -> (-13.07, 10.5628)
  line L581 (-14.2154, 13.3626) -> (-14.2375, 13.4453)
  line L582 (17.5782, 1.4445) -> (17.6003, 1.5272)
  line L583 (17.6003, 1.5272) -> (17.5782, 1.6098)
  line L584 (17.5782, 1.6098) -> (17.5177, 1.6703)
  line L585 (17.5177, 1.6703) -> (17.435, 1.6925)
  line L586 (17.435, 1.6925) -> (17.3523, 1.6703)
  line L587 (17.3523, 1.6703) -> (17.2918, 1.6098)
  line L588 (3.0162, 1.7817) -> (3.0384, 1.699)
  line L589 (17.2918, 1.6098) -> (17.2697, 1.5272)
  line L590 (17.2697, 1.5272) -> (17.2918, 1.4445)
  line L591 (3.0384, 1.8643) -> (3.0162, 1.7817)
  line L592 (17.2918, 1.4445) -> (17.3523, 1.384)
  line L593 (3.0989, 1.9249) -> (3.0384, 1.8643)
  line L594 (3.2642, 1.6385) -> (3.3248, 1.699)
  line L595 (3.3248, 1.699) -> (3.3469, 1.7817)
  line L596 (3.2642, 1.9249) -> (3.1816, 1.947)
  line L597 (3.3469, 1.7817) -> (3.3248, 1.8643)
  line L598 (3.3248, 1.8643) -> (3.2642, 1.9249)
  line L599 (16.3277, -9.1629) -> (16.3056, -9.0802)
  line L600 (16.3056, -9.0802) -> (16.245, -9.0197)
  line L601 (16.245, -9.0197) -> (16.1624, -8.9976)
  line L602 (16.1624, -8.9976) -> (16.0797, -9.0197)
  line L603 (16.0192, -9.2456) -> (16.0797, -9.3061)
  line L604 (16.0797, -9.0197) -> (16.0192, -9.0802)
  line L605 (16.0192, -9.0802) -> (15.997, -9.1629)
  line L606 (15.997, -9.1629) -> (16.0192, -9.2456)
  line L607 (13.3626, -14.9789) -> (13.2799, -15.0011)
  line L608 (3.856, -2.1635) -> (3.8338, -2.0808)
  line L609 (3.8338, -2.0808) -> (3.7733, -2.0203)
  line L610 (13.2194, -15.2269) -> (13.2799, -15.2875)
  line L611 (13.2799, -15.0011) -> (13.2194, -15.0616)
  line L612 (13.2194, -15.0616) -> (13.1972, -15.1443)
  line L613 (13.1972, -15.1443) -> (13.2194, -15.2269)
  line L614 (13.2799, -15.2875) -> (13.3626, -15.3096)
  line L615 (13.3626, -15.3096) -> (13.4453, -15.2875)
  line L616 (13.4453, -15.2875) -> (13.5058, -15.2269)
  line L617 (13.5058, -15.2269) -> (13.5279, -15.1443)
  line L618 (13.5279, -15.1443) -> (13.5058, -15.0616)
  line L619 (13.4453, -15.0011) -> (13.3626, -14.9789)
  line L620 (-14.8517, 7.254) -> (-14.8738, 7.3366)
  line L621 (-14.8738, 7.3366) -> (-14.9343, 7.3972)
  line L622 (-14.9343, 7.3972) -> (-15.017, 7.4193)
  line L623 (-15.017, 7.4193) -> (-15.0997, 7.3972)
  line L624 (-15.0997, 7.3972) -> (-15.1602, 7.3366)
  line L625 (-15.1602, 7.3366) -> (-15.1823, 7.254)
  line L626 (-14.8517, 4.7087) -> (-14.8738, 4.7914)
  line L627 (-14.8738, 4.7914) -> (-14.9343, 4.8519)
  line L628 (-14.9343, 4.8519) -> (-15.017, 4.8741)
  line L629 (-15.017, 4.8741) -> (-15.0997, 4.8519)
  line L630 (-15.1602, 4.6261) -> (-15.0997, 4.5655)
  line L631 (-15.0997, 4.8519) -> (-15.1602, 4.7914)
  line L632 (-15.1602, 4.7914) -> (-15.1823, 4.7087)
  line L633 (-15.1823, 4.7087) -> (-15.1602, 4.6261)
  line L634 (-15.0997, 4.5655) -> (-15.017, 4.5434)
  line L635 (-15.017, 4.5434) -> (-14.9343, 4.5655)
  line L636 (-14.9343, 4.5655) -> (-14.8738, 4.6261)
  line L637 (-14.8738, 4.6261) -> (-14.8517, 4.7087)
  line L638 (13.5058, 2.0808) -> (13.5279, 2.1635)
  line L639 (13.3626, 1.9981) -> (13.4453, 2.0203)
  line L640 (13.4453, 2.0203) -> (13.5058, 2.0808)
  line L641 (-7.5085, 7.763) -> (-7.5426, 7.8903)
  line L642 (-7.5426, 7.8903) -> (-7.6358, 7.9835)
  line L643 (-7.6358, 7.9835) -> (-7.763, 8.0176)
  line L644 (-7.763, 8.0176) -> (-7.8903, 7.9835)
  line L645 (-7.8903, 7.9835) -> (-7.9835, 7.8903)
  line L646 (-7.9835, 7.8903) -> (-8.0176, 7.763)
  line L647 (-8.0176, 7.763) -> (-7.9835, 7.6358)
  line L648 (-7.9835, 7.6358) -> (-7.8903, 7.5426)
  line L649 (-7.8903, 7.5426) -> (-7.763, 7.5085)
  line L650 (-7.763, 7.5085) -> (-7.6358, 7.5426)
  line L651 (-11.6922, 17.5177) -> (-11.7528, 17.5782)
  line L652 (12.3445, -12.1791) -> (12.2618, -12.2013)
  line L653 (-12.7103, 17.3523) -> (-12.6882, 17.435)
  line L654 (-13.5344, -15.7647) -> (-13.6171, -15.7425)
  line L655 (-12.6882, 17.435) -> (-12.7103, 17.5177)
  line L656 (-15.0261, -16.1624) -> (-14.8897, -15.6533)
  line L657 (8.0176, 15.3096) -> (7.9349, 15.2875)
  line L658 (-7.8903, -7.5426) -> (-7.9835, -7.6358)
  line L659 (-0.7255, 17.435) -> (-0.7476, 17.5177)
  line L660 (7.8522, 15.1443) -> (7.8744, 15.0616)
  line L661 (-12.7709, 17.2918) -> (-12.7103, 17.3523)
  line L662 (7.8744, 15.2269) -> (7.8522, 15.1443)
  line L663 (-13.4518, -15.9078) -> (-13.4739, -15.8252)
  line L664 (-17.435, -14.5971) -> (-17.5177, -14.6193)
  line L665 (-17.435, 11.7463) -> (-17.5177, 11.7241)
  line L666 (-15.9078, 12.9427) -> (-15.8252, 12.9649)
  line L667 (-13.6171, -15.7425) -> (-13.6998, -15.7647)
  line L668 (-14.8738, 7.1713) -> (-14.8517, 7.254)
  line L669 (-15.7965, -13.4453) -> (-15.736, -13.5058)
  line L670 (-15.736, -13.5058) -> (-15.6533, -13.5279)
  line L671 (-12.599, 13.2734) -> (-12.6817, 13.2513)
  line L672 (-1.2886, 5.6442) -> (-1.228, 5.5836)
  line L673 (-12.7422, 13.1907) -> (-12.7644, 13.1081)
  line L674 (-17.2918, 6.8276) -> (-17.3523, 6.8881)
  line L675 (-2.6394, 17.0995) -> (-2.3825, 17.3276)
  line L676 (-12.7644, 13.1081) -> (-12.7422, 13.0254)
  line L677 (-16.4169, 5.307) -> (-16.3342, 5.3291)
  line L678 (-13.1763, 15.2715) -> (-13.3626, 15.4579)
  line L679 (-11.7528, 17.5782) -> (-11.8354, 17.6003)
  line L680 (-11.9786, 17.5177) -> (-12.0008, 17.435)
  line L681 (14.7784, 2.3353) -> (14.8006, 2.418)
  line L682 (-17.435, 6.9103) -> (-17.5177, 6.8881)
  line L683 (-13.1081, 15.017) -> (-13.1763, 15.2715)
  line L684 (1.6925, 3.5634) -> (1.6703, 3.646)
  line L685 (-12.4558, 13.0254) -> (-12.4337, 13.1081)
  line L686 (-11.9181, 17.5782) -> (-11.9786, 17.5177)
  line L687 (-12.5163, 12.9649) -> (-12.4558, 13.0254)
  line L688 (-12.599, 12.9427) -> (-12.5163, 12.9649)
  line L689 (-12.6817, 12.9649) -> (-12.599, 12.9427)
  line L690 (-12.7422, 13.0254) -> (-12.6817, 12.9649)
  line L691 (-1.3999, 8.6919) -> (-1.4826, 8.6698)
  line L692 (-13.6171, 14.508) -> (-13.3626, 14.5762)
  line L693 (-8.1218, 18.4531) -> (-13.3626, 18.4531)
  line L694 (-16.5601, 5.3896) -> (-16.4996, 5.3291)
  line L695 (-8.1218, 18.4531) -> (-7.9701, 18.1449)
  line L696 (-7.9701, 18.1449) -> (-7.7893, 17.8528)
  line L697 (-7.7893, 17.8528) -> (-7.5812, 17.5795)
  line L698 (-7.5812, 17.5795) -> (-7.3475, 17.3276)
  line L699 (-7.3475, 17.3276) -> (-7.0907, 17.0995)
  line L700 (-7.0907, 17.0995) -> (-6.813, 16.8973)
  line L701 (-6.813, 16.8973) -> (-6.517, 16.7229)
  line L702 (-6.517, 16.7229) -> (-6.2056, 16.5779)
  line L703 (-6.2056, 16.5779) -> (-5.8816, 16.4637)
  line L704 (-5.8816, 16.4637) -> (-5.5481, 16.3813)
  line L705 (-5.5481, 16.3813) -> (-5.2082, 16.3316)
  line L706 (-5.2082, 16.3316) -> (-4.865, 16.315)
  line L707 (-4.865, 16.315) -> (-4.5219, 16.3316)
  line L708 (-4.5219, 16.3316) -> (-4.182, 16.3813)
  line L709 (-4.182, 16.3813) -> (-3.8485, 16.4637)
  line L710 (-3.8485, 16.4637) -> (-3.5245, 16.5779)
  line L711 (-3.5245, 16.5779) -> (-3.2131, 16.7229)
  line L712 (-3.2131, 16.7229) -> (-2.9171, 16.8973)
  line L713 (-2.9171, 16.8973) -> (-2.6394, 17.0995)
  line L714 (-2.3825, 17.3276) -> (-2.1489, 17.5795)
  line L715 (-14.6352, 15.6533) -> (-14.7716, 16.1624)
  line L716 (-14.7716, 16.1624) -> (-15.1443, 16.535)
  line L717 (-15.1443, 16.535) -> (-15.6533, 16.6714)
  line L718 (-15.6533, 16.6714) -> (-16.1624, 16.535)
  line L719 (-16.1624, 16.535) -> (-16.535, 16.1624)
  line L720 (-16.535, 16.1624) -> (-16.6714, 15.6533)
  line L721 (-16.6714, 15.6533) -> (-16.535, 15.1443)
  line L722 (-16.535, 15.1443) -> (-16.1624, 14.7716)
  line L723 (-16.1624, 14.7716) -> (-15.6533, 14.6352)
  line L724 (-15.6533, 14.6352) -> (-15.1443, 14.7716)
  line L725 (-15.1443, 14.7716) -> (-14.7716, 15.1443)
  line L726 (-14.7716, 15.1443) -> (-14.6352, 15.6533)
  line L727 (16.6714, -15.6533) -> (16.535, -15.1443)
  line L728 (16.535, -15.1443) -> (16.1624, -14.7716)
  line L729 (16.1624, -14.7716) -> (15.6533, -14.6352)
  line L730 (15.6533, -14.6352) -> (15.1443, -14.7716)
  line L731 (15.1443, -14.7716) -> (14.7716, -15.1443)
  line L732 (14.7716, -15.1443) -> (14.6352, -15.6533)
  line L733 (14.6352, -15.6533) -> (14.7716, -16.1624)
  line L734 (14.7716, -16.1624) -> (15.1443, -16.535)
  line L735 (-14.8897, -15.6533) -> (-15.0261, -15.1443)
  line L736 (-15.0261, -15.1443) -> (-15.3988, -14.7716)
  line L737 (-15.3988, -14.7716) -> (-15.9078, -14.6352)
  line L738 (-15.9078, -14.6352) -> (-16.4169, -14.7716)
  line L739 (-16.4169, -14.7716) -> (-16.7895, -15.1443)
  line L740 (-16.7895, -15.1443) -> (-16.9259, -15.6533)
  line L741 (-16.9259, -15.6533) -> (-16.7895, -16.1624)
  line L742 (-16.7895, -16.1624) -> (-16.4169, -16.535)
  line L743 (-16.4169, -16.535) -> (-15.9078, -16.6714)
  line L744 (-15.9078, -16.6714) -> (-15.3988, -16.535)
  line L745 (16.1624, -2.927) -> (16.026, -2.418)
  line L746 (16.026, -2.418) -> (15.6533, -2.0453)
  line L747 (15.6533, -2.0453) -> (15.1443, -1.9089)
  line L748 (15.1443, -1.9089) -> (14.6352, -2.0453)
  line L749 (14.6352, -2.0453) -> (14.2626, -2.418)
  line L750 (14.2626, -2.418) -> (14.1262, -2.927)
  line L751 (14.1262, -2.927) -> (14.2626, -3.4361)
  line L752 (14.2626, -3.4361) -> (14.6352, -3.8087)
  line L753 (14.6352, -3.8087) -> (15.1443, -3.9451)
  line L754 (15.1443, -3.9451) -> (15.6533, -3.8087)
  line L755 (15.6533, -3.8087) -> (16.026, -3.4361)
  line L756 (-13.6171, 15.5261) -> (-13.8716, 15.4579)
  line L757 (-13.8716, 15.4579) -> (-14.058, 15.2715)
  line L758 (-14.058, 15.2715) -> (-14.1262, 15.017)
  line L759 (-14.1262, 15.017) -> (-14.058, 14.7625)
  line L760 (-14.058, 14.7625) -> (-13.8716, 14.5762)
  line L761 (-13.8716, 14.5762) -> (-13.6171, 14.508)
  line L762 (-13.3626, 14.5762) -> (-13.1763, 14.7625)
  line L763 (-13.1763, 14.7625) -> (-13.1081, 15.017)
  line L764 (-8.0176, 16.0351) -> (-8.0858, 16.2896)
  line L765 (-8.0858, 16.2896) -> (-8.2721, 16.476)
  line L766 (-8.2721, 16.476) -> (-8.5266, 16.5442)
  line L767 (-8.5266, 16.5442) -> (-8.7811, 16.476)
  line L768 (-8.7811, 16.476) -> (-8.9675, 16.2896)
  line L769 (-8.9675, 16.2896) -> (-9.0357, 16.0351)
  line L770 (-9.0357, 16.0351) -> (-8.9675, 15.7806)
  line L771 (-8.9675, 15.7806) -> (-8.7811, 15.5943)
  line L772 (-8.7811, 15.5943) -> (-8.5266, 15.5261)
  line L773 (-8.5266, 15.5261) -> (-8.2721, 15.5943)
  line L774 (-9.0357, 13.9989) -> (-8.9675, 13.7444)
  line L775 (-8.9675, 13.7444) -> (-8.7811, 13.5581)
  line L776 (-8.7811, 13.5581) -> (-8.5266, 13.4899)
  line L777 (-8.5266, 13.4899) -> (-8.2721, 13.5581)
  line L778 (-8.2721, 13.5581) -> (-8.0858, 13.7444)
  line L779 (-8.0858, 13.7444) -> (-8.0176, 13.9989)
  line L780 (-12.4337, 13.1081) -> (-12.4558, 13.1907)
  line L781 (-12.4558, 13.1907) -> (-12.5163, 13.2513)
  line L782 (-12.5163, 13.2513) -> (-12.599, 13.2734)
  line L783 (-12.6817, 13.2513) -> (-12.7422, 13.1907)
  line L784 (-0.98, 5.7268) -> (-1.0022, 5.8095)
  line L785 (-1.0022, 5.8095) -> (-1.0627, 5.87)
  line L786 (-1.0627, 5.87) -> (-1.1454, 5.8922)
  line L787 (-1.1454, 5.8922) -> (-1.228, 5.87)
  line L788 (-1.228, 5.87) -> (-1.2886, 5.8095)
  line L789 (-1.2886, 5.8095) -> (-1.3107, 5.7268)
  line L790 (-1.3107, 5.7268) -> (-1.2886, 5.6442)
  line L791 (-1.228, 5.5836) -> (-1.1454, 5.5615)
  line L792 (-1.1454, 5.5615) -> (-1.0627, 5.5836)
  line L793 (-1.0627, 5.5836) -> (-1.0022, 5.6442)
  line L794 (-1.0022, 5.6442) -> (-0.98, 5.7268)
  line L795 (2.2015, 12.8535) -> (2.1794, 12.9362)
  line L796 (2.1794, 12.9362) -> (2.1189, 12.9967)
  line L797 (2.1189, 12.9967) -> (2.0362, 13.0189)
  line L798 (2.0362, 13.0189) -> (1.9535, 12.9967)
  line L799 (1.9535, 12.9967) -> (1.893, 12.9362)
  line L800 (1.893, 12.9362) -> (1.8709, 12.8535)
  line L801 (1.8709, 12.8535) -> (1.893, 12.7709)
  line L802 (1.893, 12.7709) -> (1.9535, 12.7103)
  line L803 (1.9535, 12.7103) -> (2.0362, 12.6882)
  line L804 (2.0362, 12.6882) -> (2.1189, 12.7103)
  line L805 (2.1189, 12.7103) -> (2.1794, 12.7709)
  line L806 (2.1794, 12.7709) -> (2.2015, 12.8535)
  line L807 (-8.8703, 17.435) -> (-8.8925, 17.5177)
  line L808 (-8.8925, 17.5177) -> (-8.953, 17.5782)
  line L809 (-8.953, 17.5782) -> (-9.0357, 17.6003)
  line L810 (-9.1183, 17.5782) -> (-9.1788, 17.5177)
  line L811 (-9.1788, 17.5177) -> (-9.201, 17.435)
  line L812 (-9.201, 17.435) -> (-9.1788, 17.3523)
  line L813 (-9.1788, 17.3523) -> (-9.1183, 17.2918)
  line L814 (-9.1183, 17.2918) -> (-9.0357, 17.2697)
  line L815 (-9.0357, 17.2697) -> (-8.953, 17.2918)
  line L816 (-8.953, 17.2918) -> (-8.8925, 17.3523)
  line L817 (-8.8925, 17.3523) -> (-8.8703, 17.435)
  line L818 (11.1832, 12.5163) -> (11.2437, 12.4558)
  line L819 (-11.6701, 17.435) -> (-11.6922, 17.5177)
  line L820 (-12.0008, 17.435) -> (-11.9786, 17.3523)
  line L821 (-11.9786, 17.3523) -> (-11.9181, 17.2918)
  line L822 (-11.9181, 17.2918) -> (-11.8354, 17.2697)
  line L823 (-11.6922, 17.3523) -> (-11.6701, 17.435)
  line L824 (10.5628, 13.2734) -> (10.4801, 13.2513)
  line L825 (10.4801, 13.2513) -> (10.4196, 13.1907)
  line L826 (8.1607, 15.2269) -> (8.1002, 15.2875)
  line L827 (8.1002, 15.2875) -> (8.0176, 15.3096)
  line L828 (7.9349, 15.2875) -> (7.8744, 15.2269)
  line L829 (7.8744, 15.0616) -> (7.9349, 15.0011)
  line L830 (7.9349, 15.0011) -> (8.0176, 14.9789)
  line L831 (8.0176, 14.9789) -> (8.1002, 15.0011)
  line L832 (8.1002, 15.0011) -> (8.1607, 15.0616)
  line L833 (8.1607, 15.0616) -> (8.1829, 15.1443)
  line L834 (-1.2345, 16.4169) -> (-1.2567, 16.4996)
  line L835 (-1.2567, 16.4996) -> (-1.3172, 16.5601)
  line L836 (-1.3172, 16.5601) -> (-1.3999, 16.5822)
  line L837 (-1.3999, 16.5822) -> (-1.4826, 16.5601)
  line L838 (-1.4826, 16.5601) -> (-1.5431, 16.4996)
  line L839 (-1.5431, 16.4996) -> (-1.5652, 16.4169)
  line L840 (-1.5652, 16.4169) -> (-1.5431, 16.3342)
  line L841 (-1.5431, 16.3342) -> (-1.4826, 16.2737)
  line L842 (-1.4826, 16.2737) -> (-1.3999, 16.2516)
  line L843 (-1.3999, 16.2516) -> (-1.3172, 16.2737)
  line L844 (-1.3172, 16.2737) -> (-1.2567, 16.3342)
  line L845 (-1.2567, 16.3342) -> (-1.2345, 16.4169)
  line L846 (13.6552, 12.4718) -> (13.633, 12.5544)
  line L847 (13.633, 12.5544) -> (13.5725, 12.6149)
  line L848 (13.5725, 12.6149) -> (13.4899, 12.6371)
  line L849 (13.4899, 12.6371) -> (13.4072, 12.6149)
  line L850 (13.4072, 12.6149) -> (13.3467, 12.5544)
  line L851 (13.3467, 12.5544) -> (13.3245, 12.4718)
  line L852 (13.3245, 12.4718) -> (13.3467, 12.3891)
  line L853 (13.3467, 12.3891) -> (13.4072, 12.3286)
  line L854 (13.4072, 12.3286) -> (13.4899, 12.3064)
  line L855 (13.4899, 12.3064) -> (13.5725, 12.3286)
  line L856 (13.5725, 12.3286) -> (13.633, 12.3891)
  line L857 (13.633, 12.3891) -> (13.6552, 12.4718)
  line L858 (14.6733, 11.4536) -> (14.6511, 11.5363)
  line L859 (14.6511, 11.5363) -> (14.5906, 11.5968)
  line L860 (14.5906, 11.5968) -> (14.508, 11.619)
  line L861 (14.508, 11.619) -> (14.4253, 11.5968)
  line L862 (14.4253, 11.5968) -> (14.3648, 11.5363)
  line L863 (14.3648, 11.5363) -> (14.3426, 11.4536)
  line L864 (14.3426, 11.4536) -> (14.3648, 11.371)
  line L865 (14.3648, 11.371) -> (14.4253, 11.3105)
  line L866 (14.4253, 11.3105) -> (14.508, 11.2883)
  line L867 (14.508, 11.2883) -> (14.5906, 11.3105)
  line L868 (14.5906, 11.3105) -> (14.6511, 11.371)
  line L869 (14.6511, 11.371) -> (14.6733, 11.4536)
  line L870 (8.4374, 17.435) -> (8.4153, 17.5177)
  line L871 (8.4153, 17.5177) -> (8.3548, 17.5782)
  line L872 (8.3548, 17.5782) -> (8.2721, 17.6003)
  line L873 (8.2721, 17.6003) -> (8.1894, 17.5782)
  line L874 (8.1894, 17.5782) -> (8.1289, 17.5177)
  line L875 (8.1289, 17.5177) -> (8.1067, 17.435)
  line L876 (8.1067, 17.435) -> (8.1289, 17.3523)
  line L877 (8.1289, 17.3523) -> (8.1894, 17.2918)
  line L878 (8.1894, 17.2918) -> (8.2721, 17.2697)
  line L879 (8.2721, 17.2697) -> (8.3548, 17.2918)
  line L880 (8.3548, 17.2918) -> (8.4153, 17.3523)
  line L881 (8.4153, 17.3523) -> (8.4374, 17.435)
  line L882 (5.7649, 17.435) -> (5.7428, 17.5177)
  line L883 (5.7428, 17.5177) -> (5.6822, 17.5782)
  line L884 (5.6822, 17.5782) -> (5.5996, 17.6003)
  line L885 (5.5996, 17.6003) -> (5.5169, 17.5782)
  line L886 (5.5169, 17.5782) -> (5.4564, 17.5177)
  line L887 (5.4564, 17.5177) -> (5.4342, 17.435)
  line L888 (5.4342, 17.435) -> (5.4564, 17.3523)
  line L889 (5.4564, 17.3523) -> (5.5169, 17.2918)
  line L890 (5.5169, 17.2918) -> (5.5996, 17.2697)
  line L891 (5.5996, 17.2697) -> (5.6822, 17.2918)
  line L892 (5.6822, 17.2918) -> (5.7428, 17.3523)
  line L893 (5.7428, 17.3523) -> (5.7649, 17.435)
  line L894 (6.9103, 17.435) -> (6.8881, 17.5177)
  line L895 (6.8881, 17.5177) -> (6.8276, 17.5782)
  line L896 (6.8276, 17.5782) -> (6.7449, 17.6003)
  line L897 (6.7449, 17.6003) -> (6.6623, 17.5782)
  line L898 (6.6623, 17.5782) -> (6.6017, 17.5177)
  line L899 (6.6017, 17.5177) -> (6.5796, 17.435)
  line L900 (6.5796, 17.435) -> (6.6017, 17.3523)
  line L901 (6.6017, 17.3523) -> (6.6623, 17.2918)
  line L902 (6.6623, 17.2918) -> (6.7449, 17.2697)
  line L903 (6.7449, 17.2697) -> (6.8276, 17.2918)
  line L904 (6.8276, 17.2918) -> (6.8881, 17.3523)
  line L905 (6.8881, 17.3523) -> (6.9103, 17.435)
  line L906 (17.6003, 8.0176) -> (17.5782, 8.1002)
  line L907 (17.5782, 8.1002) -> (17.5177, 8.1607)
  line L908 (17.5177, 8.1607) -> (17.435, 8.1829)
  line L909 (17.435, 8.1829) -> (17.3523, 8.1607)
  line L910 (17.3523, 8.1607) -> (17.2918, 8.1002)
  line L911 (17.2918, 8.1002) -> (17.2697, 8.0176)
  line L912 (17.2697, 8.0176) -> (17.2918, 7.9349)
  line L913 (17.2918, 7.9349) -> (17.3523, 7.8744)
  line L914 (17.3523, 7.8744) -> (17.435, 7.8522)
  line L915 (17.435, 7.8522) -> (17.5177, 7.8744)
  line L916 (17.5177, 7.8744) -> (17.5782, 7.9349)
  line L917 (17.5782, 7.9349) -> (17.6003, 8.0176)
  line L918 (17.6003, 5.9813) -> (17.5782, 6.064)
  line L919 (17.5782, 6.064) -> (17.5177, 6.1245)
  line L920 (17.5177, 6.1245) -> (17.435, 6.1467)
  line L921 (17.435, 6.1467) -> (17.3523, 6.1245)
  line L922 (17.3523, 6.1245) -> (17.2918, 6.064)
  line L923 (17.2918, 6.064) -> (17.2697, 5.9813)
  line L924 (17.2697, 5.9813) -> (17.2918, 5.8987)
  line L925 (17.2918, 5.8987) -> (17.3523, 5.8382)
  line L926 (17.3523, 5.8382) -> (17.435, 5.816)
  line L927 (17.435, 5.816) -> (17.5177, 5.8382)
  line L928 (17.5177, 5.8382) -> (17.5782, 5.8987)
  line L929 (17.5782, 5.8987) -> (17.6003, 5.9813)
  line L930 (17.6003, 0.3818) -> (17.5782, 0.4645)
  line L931 (17.5782, 0.4645) -> (17.5177, 0.525)
  line L932 (17.5177, 0.525) -> (17.435, 0.5471)
  line L933 (17.435, 0.5471) -> (17.3523, 0.525)
  line L934 (17.3523, 0.525) -> (17.2918, 0.4645)